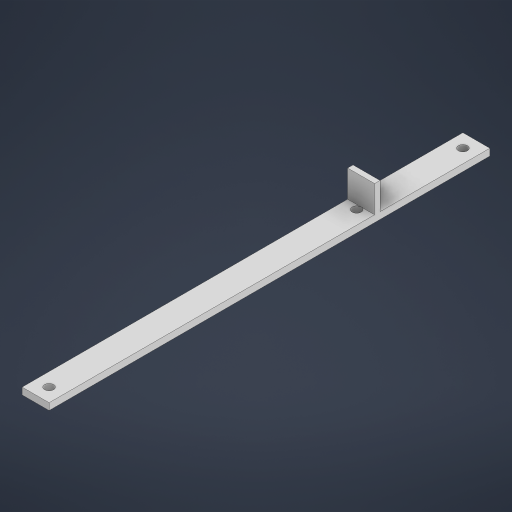
# Autodesk Inventor part: mock piston (single acting)
Saved by Autodesk Inventor 2024 (Build 280153000, 153)
## iProperties
Created: 2024-02-12
Part Number: mock piston (single acting)
Material: Generic
Document SubType Name: Modeling
Designer: elite
Density: 1 g/cm^3
Appearance: Default
Author: elite
Autodesk Inventor part; units mm, degrees
ref_plane "YZ Plane" through (0, 0, 0) normal (1, 0, 0) x (0, 1, 0)
ref_plane "XZ Plane" through (0, 0, 0) normal (0, 1, 0) x (-1, 0, 0)
ref_plane "XY Plane" through (0, 0, 0) normal (0, 0, 1) x (1, 0, 0)
sketch "Sketch1" plane through (0, 0, 0) normal (0, 1, 0) x (-1, 0, 0)
  line L0 (0, 0) -> (12.7, 0)
  line L1 (12.7, 0) -> (12.7, -151.13)
  line L2 (12.7, -151.13) -> (0, -151.13)
  line L3 (0, -151.13) -> (0, 0)
  line L4 (6.35, 0) -> (6.35, -6.35)
  circle A0 centre (6.35, -6.35) radius 2.1082
  circle A1 centre (6.35, -151.13) radius 2.1082
  line L5 (6.35, -151.13) -> (6.35, -201.13)
  circle A2 centre (6.35, -201.13) radius 2.1082
  line L6 (6.35, -201.13) -> (0, -201.13)
  line L7 (0, -201.13) -> (0, -207.48)
  line L8 (0, -207.48) -> (12.7, -207.48)
  line L9 (12.7, -207.48) -> (12.7, -151.13)
  line L10 (12.7, -151.13) -> (0, -151.13)
  line L11 (0, -151.13) -> (0, -207.48)
  point P0 (0, -151.13)
  dimension "d0" = 12.7
  dimension "d2" = 6.35
  dimension "d3" = 4.2164
  dimension "d4" = 144.78
  dimension "d5" = 4.2164
  dimension "d6" = 50
  dimension "d7" = 4.2164
  dimension "d8" = 6.35
  constraints: 24 end point, 4 parallel, 3 centre point, 3 horizontal, 3 perpendicular, 2 coincident, 2 midpoint, 2 vertical
  measures "d0" distance of L1.end L2.end
  measures "d2" distance of L4.start L4.end
  measures "d3" diameter of A0
  measures "d4" distance from line of L2 L4.end
  measures "d5" diameter of A1
  measures "d6" distance of L5.start L5.end
  measures "d7" diameter of A2
  measures "d8" distance of L6.end L7.end
extrude "Extrusion1" add sketch "Sketch1" along normal blind 3.175 contours L0 L1 L2 A1 L3 | L2 A1 L5 A2 L6 L11 | L6 A2 L5 A1 L2 L9 L8 L7
sketch "Sketch2" plane through (0, 3.175, 0) normal (0, 1, 0) x (1, 0, 0)
  circle A0 centre (-6.35, 151.13) radius 2.1082 projected
  line L0 (-6.35, 153.2382) -> (0, 153.2382)
  line L1 (-6.35, 153.2382) -> (-12.7, 153.2382)
  line L2 (0, 0) -> (0, 207.48) projected
  line L3 (-12.7, 153.2382) -> (0, 153.2382)
  line L4 (0, 153.2382) -> (0, 155.7782)
  line L5 (0, 155.7782) -> (-12.7, 155.7782)
  line L6 (-12.7, 155.7782) -> (-12.7, 153.2382)
  dimension "d11" = 6.35
  dimension "d12" = 2.54
  constraints: 12 end point, 5 horizontal, 2 parallel, 1 perpendicular, 1 point on line, 1 vertical alignment, 1 other
  measures "d11" distance of L0.start L1.end
  measures "d12" distance of L5.end L1.end
extrude "Extrusion2" add sketch "Sketch2" along normal blind 12.7 contours L1 L6 L5 L2 L0
body "Solid1"
